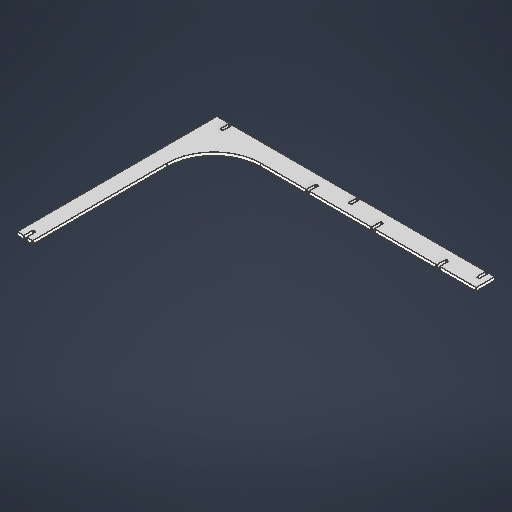
# Autodesk Inventor part: slats_back_under
Saved by Autodesk Inventor 2027.1 (Build 311270010, 270A)
## iProperties
Created: 2025-09-12
Part Number: slats_back_under
Material: Foam Core Board
Document SubType Name: Modeling
Designer: Nick
Density: 0.141998 g/cm^3
Appearance: Default(1)
Mass: 15.1466 g
Surface Area: 511.354 cm^2
Volume: 106.668 cm^3
Author: Nick
Autodesk Inventor part; units mm, degrees
ref_plane "YZ Plane" through (0, 0, 0) normal (1, 0, 0) x (0, 1, 0)
ref_plane "XZ Plane" through (0, 0, 0) normal (0, 1, 0) x (-1, 0, 0)
ref_plane "XY Plane" through (0, 0, 0) normal (0, 0, 1) x (1, 0, 0)
sketch "Sketch1" plane through (0, 0, 0) normal (0, 1, 0) x (-1, 0, 0)
  line L0 (0, 0) -> (435, 0)
  line L1 (435, 0) -> (435, -30)
  line L2 (435, -30) -> (0, -30)
  line L3 (0, -30) -> (0, 0)
  dimension "d0" = 435
  dimension "d1" = 30
  constraints: 8 end point, 2 parallel, 1 horizontal, 1 perpendicular
  measures "d0" distance of L1.end L2.end
  measures "d1" distance of L0.end L1.end
extrude "Extrusion1" add sketch "Sketch1" along normal blind 5
sketch "Sketch2" plane through (0, 5, 0) normal (0, 1, 0) x (1, 0, 0)
  line L0 (0, 30) -> (-435, 30) projected
  line L1 (-435, 30) -> (-425, 30)
  line L2 (-425, 30) -> (-420.5, 30)
  line L3 (-420.5, 30) -> (-420.5, 15)
  line L4 (-420.5, 15) -> (-425, 15)
  line L5 (-425, 15) -> (-425, 30)
  line L6 (-420.5, 30) -> (-219.75, 30)
  line L7 (-219.75, 30) -> (-215.25, 30)
  line L8 (-215.25, 30) -> (-215.25, 15)
  line L9 (-215.25, 15) -> (-219.75, 15)
  line L10 (-219.75, 15) -> (-219.75, 30)
  line L11 (-215.25, 30) -> (-14.5, 30)
  line L12 (-14.5, 30) -> (-10, 30)
  line L13 (-10, 30) -> (-10, 15)
  line L14 (-10, 15) -> (-14.5, 15)
  line L15 (-14.5, 15) -> (-14.5, 30)
  point P0 (0, 0)
  dimension "d4" = 10
  dimension "d5" = 4.5
  dimension "d6" = 15
  dimension "d7" = 200.75
  dimension "d8" = 4.5
  dimension "d9" = 15
  dimension "d10" = 200.75
  dimension "d11" = 4.5
  dimension "d12" = 15
  constraints: 30 end point, 6 parallel, 3 horizontal, 3 perpendicular, 3 point on line
  measures "d4" distance of L0.end L1.end
  measures "d5" distance of L3.end L4.end
  measures "d6" distance of L2.end L3.end
  measures "d7" distance of L2.end L6.end
  measures "d8" distance of L8.end L9.end
  measures "d9" distance of L7.end L8.end
  measures "d10" distance of L7.end L11.end
  measures "d11" distance of L13.end L14.end
  measures "d12" distance of L12.end L13.end
extrude "Extrusion2" cut sketch "Sketch2" against normal blind 5
sketch "Sketch3" plane through (0, 5, 0) normal (0, 1, 0) x (1, 0, 0)
  line L0 (-435, 30) -> (-435, 0) projected
  line L1 (-435, 30) -> (-445, 30)
  line L2 (-445, 30) -> (-445, -290)
  line L3 (-445, -290) -> (-435, -290)
  line L4 (-435, -290) -> (-435, 30)
  line L5 (-435, -290) -> (-420, -290)
  line L6 (-420, -290) -> (-420, 15)
  line L7 (-420, 15) -> (-435, 15)
  line L8 (-435, 15) -> (-435, -290)
  point P0 (0, 0)
  dimension "d15" = 10
  dimension "d16" = 320
  dimension "d17" = 15
  dimension "d18" = 305
  constraints: 16 end point, 4 parallel, 2 horizontal, 2 perpendicular
  measures "d15" distance of L3.end L2.end
  measures "d16" distance of L1.end L2.end
  measures "d17" distance of L7.end L6.end
  measures "d18" distance of L5.end L6.end
extrude "Extrusion3" add sketch "Sketch3" against normal blind 5
fillet "Fillet1" radius 75 1 edges at (-420, 2.5, 0)
sketch "Sketch4" plane through (0, 5, 0) normal (0, 1, 0) x (1, 0, 0)
  line L0 (-10, 15) -> (-14.5, 15) projected
  line L1 (-14.5, 15) -> (-58.5, 15)
  line L2 (-345, 0) -> (0, 0) projected
  line L3 (-58.5, 15) -> (-63, 15)
  line L4 (-63, 15) -> (-63, 0)
  line L5 (-63, 0) -> (-58.5, 0)
  line L6 (-58.5, 0) -> (-58.5, 15)
  line L7 (-63, 0) -> (-110.75, 0)
  line L8 (-110.75, 0) -> (-115.25, 0)
  line L9 (-115.25, 0) -> (-115.25, 15)
  line L10 (-115.25, 15) -> (-110.75, 15)
  line L11 (-110.75, 15) -> (-110.75, 0)
  line L12 (-115.25, 0) -> (-163, 0)
  line L13 (-163, 0) -> (-215.25, 0)
  line L14 (-215.25, 0) -> (-219.75, 0)
  line L15 (-163, 0) -> (-167.5, 0)
  line L16 (-167.5, 0) -> (-167.5, 15)
  line L17 (-167.5, 15) -> (-163, 15)
  line L18 (-163, 15) -> (-163, 0)
  line L19 (-217.5, 0) -> (-217.5, 32.2246)
  line L20 (-372, 0) -> (-324.25, 0)
  line L21 (-324.25, 0) -> (-319.75, 0)
  line L22 (-319.75, 0) -> (-319.75, 15)
  line L23 (-319.75, 15) -> (-324.25, 15)
  line L24 (-324.25, 15) -> (-324.25, 0)
  line L25 (-319.75, 0) -> (-272, 0)
  line L26 (-272, 0) -> (-267.5, 0)
  line L27 (-267.5, 0) -> (-267.5, 15)
  line L28 (-267.5, 15) -> (-272, 15)
  line L29 (-272, 15) -> (-272, 0)
  line L30 (-372, 0) -> (-376.5, 0)
  line L31 (-376.5, 0) -> (-376.5, 30)
  line L32 (-376.5, 30) -> (-372, 30)
  line L33 (-372, 30) -> (-372, 0)
  line L34 (-376.5, 30) -> (-372, 30)
  line L35 (-372, 30) -> (-372, 15)
  line L36 (-372, 15) -> (-376.5, 15)
  line L37 (-376.5, 15) -> (-376.5, 30)
  dimension "d22" = 44
  dimension "d23" = 4.5
  dimension "d24" = 47.75
  dimension "d25" = 4.5
  dimension "d26" = 15
  dimension "d27" = 47.75
  dimension "d28" = 52.25
  dimension "d29" = 4.5
  dimension "d30" = 4.5
  dimension "d31" = 15
  dimension "d38" = 4.5
  dimension "d39" = 30
  constraints: 72 end point, 10 parallel, 9 symmetric about line, 6 horizontal, 5 perpendicular, 5 point on line, 2 midpoint, 1 vertical
  measures "d22" distance of L0.end L1.end
  measures "d23" distance of L5.end L4.end
  measures "d24" distance of L4.end L7.end
  measures "d25" distance of L9.end L10.end
  measures "d26" distance of L8.end L9.end
  measures "d27" distance of L8.end L12.end
  measures "d28" distance of L12.end L13.end
  measures "d29" distance of L13.end L14.end
  measures "d30" distance of L16.end L17.end
  measures "d31" distance of L15.end L16.end
  measures "d38" distance of L31.end L32.end
  measures "d39" distance of L30.end L31.end
extrude "Extrusion4" cut sketch "Sketch4" against normal blind 5 contours L4 L3 L6 L2 | L16 L17 L18 L2 | L29 L28 L27 L2
sketch "Sketch6" plane through (0, 5, 0) normal (0, 1, 0) x (1, 0, 0)
  line L0 (-420, -290) -> (-429.75, -290)
  line L1 (-445, -290) -> (-420, -290) projected
  line L2 (-429.75, -290) -> (-434.25, -290)
  line L3 (-434.25, -290) -> (-434.25, -275)
  line L4 (-434.25, -275) -> (-429.75, -275)
  line L5 (-429.75, -275) -> (-429.75, -290)
  point P0 (0, 0)
  dimension "d40" = 9.75
  dimension "d41" = 4.5
  dimension "d42" = 15
  constraints: 10 end point, 2 parallel, 1 horizontal, 1 perpendicular, 1 point on line
  measures "d40" distance of L0.start L0.end
  measures "d41" distance of L3.end L4.end
  measures "d42" distance of L2.end L3.end
extrude "Extrusion6" cut sketch "Sketch6" against normal blind 5
fillet "Fillet2" radius 1 31 edges at (-420, 2.5, 290) (-429.75, 2.5, 275) (-434.25, 2.5, 275) (-445, 2.5, 290) (-445, 2.5, -30) (-425, 2.5, -30) (-420.5, 2.5, -15) (-425, 2.5, -15) (-420.5, 2.5, -30) (-272, 2.5, 0) (-267.5, 2.5, 0) (-272, 2.5, -15) (-267.5, 2.5, -15) (-219.75, 2.5, -30) (-219.75, 2.5, -15) (-215.25, 2.5, -15) (-215.25, 2.5, -30) (-163, 2.5, -15) (-167.5, 2.5, -15) (-163, 2.5, 0) (-167.5, 2.5, 0) (-63, 2.5, 0) (-63, 2.5, -15) (-58.5, 2.5, -15) (-58.5, 2.5, 0) (0, 2.5, 0) (-10, 2.5, -15) (-14.5, 2.5, -15) (-14.5, 2.5, -30) (-10, 2.5, -30) (0, 2.5, -30)
body "Solid1"
